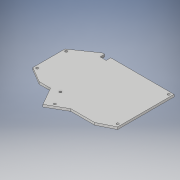
# Autodesk Inventor part: k2_base
Saved by Autodesk Inventor 2017 (Build 210142000, 142)
## iProperties
Created: 2017-02-07
Part Number: k2_base
Material: Generic
Document SubType Name: Modeling
Designer: herman
Density: 1 g/cm^3
Appearance: Default
Author: herman
Autodesk Inventor part; units mm, degrees
ref_plane "YZ Plane" through (0, 0, 0) normal (1, 0, 0) x (0, 1, 0)
ref_plane "XZ Plane" through (0, 0, 0) normal (0, 1, 0) x (-1, 0, 0)
ref_plane "XY Plane" through (0, 0, 0) normal (0, 0, 1) x (1, 0, 0)
sketch "Sketch8" plane through (0, 0, 0) normal (0, 1, 0) x (-1, 0, 0)
  line L0 (-66.1485, -125.7952) -> (27.8515, -125.7952)
  line L1 (21.8515, -51.7952) -> (8.3515, -28.4125)
  line L2 (36.8515, -51.7952) -> (21.8515, -51.7952)
  line L3 (-66.1485, -51.7952) -> (-66.1485, -125.7952)
  line L4 (8.3515, -28.4125) -> (-14.828, -41.7952)
  line L5 (36.8515, -51.7952) -> (56.8515, -63.7952)
  line L6 (56.8515, -105.7952) -> (27.8515, -125.7952)
  line L7 (56.8515, -63.7952) -> (56.8515, -105.7952)
  line L8 (-14.828, -41.7952) -> (-46.1485, -41.7952)
  line L9 (-46.1485, -41.7952) -> (-66.1485, -51.7952)
  dimension "d129" = 29
  dimension "d131" = 20
  dimension "d147" = 12
  dimension "d154" = 20
  dimension "d155" = 15
  dimension "d162" = 27
  dimension "d163" = 120
  dimension "d164" = 94
  dimension "d183" = 42
  dimension "d188" = 10
  dimension "d189" = 20
  dimension "d190" = 74
  constraints: 20 end point, 3 horizontal, 2 perpendicular, 1 vertical
  measures "d129" horizontal distance of L7.end L6.end
  measures "d131" vertical distance of L6.end L7.end
  measures "d147" vertical distance of L7.start L2.start
  measures "d154" horizontal distance of L7.start L2.start
  measures "d155" distance of L2.start L1.start
  measures "d162" distance of L1.start L1.end
  measures "d163" angle of L1 L2
  measures "d164" distance of L3.end L6.end
  measures "d183" distance of L7.start L7.end
  measures "d188" vertical distance of L3.start L8.end
  measures "d189" horizontal distance of L3.start L8.end
  measures "d190" distance of L3.start L3.end
extrude "Extrusion9" add sketch "Sketch8" along normal blind 3
sketch "Sketch9" plane through (0, 3, 0) normal (0, 1, 0) x (1, 0, 0)
  circle A0 centre (62.6485, 122.2952) radius 1.5
  circle A1 centre (-53.3515, 103.9573) radius 1.5
  circle A2 centre (-53.3515, 65.7768) radius 1.5
  circle A3 centre (-1.0082, 36.6936) radius 1.5
  circle A4 centre (-11.0082, 54.0141) radius 1.5
  line L0 (-21.8515, 51.7952) -> (-8.3515, 28.4125) projected
  line L1 (-8.3515, 28.4125) -> (14.828, 41.7952) projected
  line L2 (66.1485, 51.7952) -> (66.1485, 125.7952) projected
  line L3 (66.1485, 125.7952) -> (-27.8515, 125.7952) projected
  line L4 (-27.8515, 125.7952) -> (-56.8515, 105.7952) projected
  line L5 (-56.8515, 105.7952) -> (-56.8515, 63.7952) projected
  line L6 (-56.8515, 63.7952) -> (-36.8515, 51.7952) projected
  line L7 (-36.8515, 51.7952) -> (-21.8515, 51.7952) projected
  line L8 (-53.3515, 103.9573) -> (-26.7616, 122.2952) construction
  line L9 (-26.7616, 122.2952) -> (62.6485, 122.2952) construction
  line L10 (62.6485, 122.2952) -> (62.6485, 73.4458) construction
  line L11 (62.6485, 73.4458) -> (-7.0704, 33.1936) construction
  line L12 (-7.0704, 33.1936) -> (-19.8307, 55.2952) construction
  line L13 (-19.8307, 55.2952) -> (-35.882, 55.2952) construction
  line L14 (-35.882, 55.2952) -> (-53.3515, 65.7768) construction
  line L15 (-53.3515, 65.7768) -> (-53.3515, 103.9573) construction
  line L16 (-36.8515, 51.7952) -> (-21.8515, 51.7952) construction
  line L17 (-21.8515, 51.7952) -> (-18.8204, 53.5452) construction
  circle A5 centre (62.6485, 55.2952) radius 1.5
  line L18 (14.828, 41.7952) -> (46.1485, 41.7952) projected
  line L19 (46.1485, 41.7952) -> (66.1485, 51.7952) projected
  line L20 (-21.8515, 51.7952) -> (-8.3515, 28.4125) construction
  line L21 (-20.1015, 48.7641) -> (-11.0082, 54.0141) construction
  point P0 (0, 0)
  dimension "d135" = 3
  dimension "d136" = 3
  dimension "d137" = 3
  dimension "d165" = 3
  dimension "d166" = 3
  dimension "d169" = 3.5
  dimension "d185" = 3
  dimension "d186" = 3.5
  dimension "d187" = 3.5
  dimension "d191" = 10.5
  dimension "d192" = 7
  dimension "d193" = 3.5
  constraints: 20 end point, 6 centre point, 4 coincident, 3 point on line, 2 perpendicular, 7 other
  measures "d135" diameter of A2
  measures "d136" diameter of A1
  measures "d137" diameter of A0
  measures "d165" diameter of A3
  measures "d166" diameter of A4
  measures "d169" distance between parallel lines of L4 L8
  measures "d185" diameter of A5
  measures "d186" horizontal distance of L2.start A5.centre
  measures "d187" horizontal distance of A5.centre L2.start
  measures "d191" distance of L21.start L21.end
  measures "d192" distance of A3.centre L11.end
  measures "d193" distance between parallel lines of L17 L21
extrude "Extrusion10" cut sketch "Sketch9" against normal through all contours A0 | A1 | A2 | A3 | A4 | A5
sketch "Sketch10" plane through (0, 3, 0) normal (0, 1, 0) x (1, 0, 0)
  line L0 (-27.8515, 125.7952) -> (-56.8515, 105.7952) projected
  line L1 (66.1485, 125.7952) -> (-27.8515, 125.7952) projected
  line L2 (-24.8515, 125.7952) -> (-16.8515, 125.7952)
  line L3 (-16.8515, 125.7952) -> (-16.8515, 119.7952)
  line L4 (-16.8515, 119.7952) -> (-24.8515, 119.7952)
  line L5 (-24.8515, 119.7952) -> (-24.8515, 125.7952)
  point P0 (-17.0619, -65.3949)
  dimension "d179" = 3
  dimension "d180" = 6
  dimension "d181" = 8
  constraints: 8 end point, 2 parallel, 1 horizontal, 1 perpendicular, 1 point on line
  measures "d179" distance of L0.start L2.start
  measures "d180" distance of L4.end L2.start
  measures "d181" distance of L3.end L4.end
extrude "Extrusion11" cut sketch "Sketch10" against normal through all
body "Solid5"
